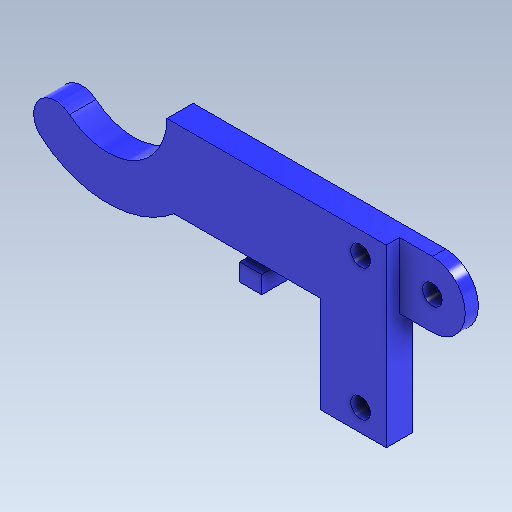
# Autodesk Inventor part: エアタンクペットボトル取付具
Saved by Autodesk Inventor 2021.3 (Build 253353010, 353A)
## iProperties
Created: 2020-02-08
Part Number: エアタンクペットボトル取付具
Material: 一般
Document SubType Name: Modeling
Designer: yuta2
Density: 1 g/cm^3
Appearance: 青 - 壁塗料 - 光沢
Author: yuta2
Autodesk Inventor part; units mm, degrees
ref_plane "YZ Plane" through (0, 0, 0) normal (1, 0, 0) x (0, 1, 0)
ref_plane "XZ Plane" through (0, 0, 0) normal (0, 1, 0) x (-1, 0, 0)
ref_plane "XY Plane" through (0, 0, 0) normal (0, 0, 1) x (1, 0, 0)
sketch "スケッチ6" plane through (0, 0, 0) normal (0, 0, 1) x (1, 0, 0)
  circle A0 centre (0, 0) radius 13.5
  circle A1 centre (0, 0) radius 23.5
  circle A2 centre (-11.8916, -14.1718) radius 5
  line L0 (0, 0) -> (-11.8916, -14.1718)
  line L1 (0, 0) -> (0, -23.5)
  line L2 (13.5, 0) -> (63.5, 0)
  line L3 (63.5, 0) -> (63.5, -18)
  line L4 (63.5, -18) -> (13.5, -18)
  line L5 (13.5, -18) -> (13.5, 0)
  line L6 (48.5, 0) -> (63.5, 0)
  line L7 (63.5, 0) -> (63.5, -40)
  line L8 (63.5, -40) -> (48.5, -40)
  line L9 (48.5, -40) -> (48.5, 0)
  point P0 (-15.1055, -18.002)
  point P1 (48.5, -18)
  point P2 (-8.6776, -10.3416)
  point P3 (23.5, 0)
  point P4 (13.3373, -19.3486)
  point P5 (13.4479, -1.1846)
  point P6 (23.5, 0)
  point P7 (15.1079, -18)
  dimension "d31" = 27
  dimension "d32" = 47
  dimension "d33" = 10
  dimension "d34" = 40
  dimension "d35" = 50
  dimension "d36" = 18
  dimension "d37" = 15
  dimension "d38" = 0
  dimension "d63" = 40
  constraints: 20 end point, 4 parallel, 2 coincident, 2 horizontal, 2 perpendicular, 2 point on line, 1 centre point, 1 vertical, 7 other
  measures "d33" diameter of A2
  measures "d34" angle of L1 L0
  measures "d35" distance of L3.end L4.end
  measures "d36" distance of L2.end L3.end
  measures "d37" distance between parallel lines of L3 L9
  measures "d38" distance between parallel lines of L2 L6
  measures "d63" distance between parallel lines of L8 L2
extrude "押し出し4" add sketch "スケッチ6" along normal blind 6 contours L5 L4 A1 L1 A0 | L2 A1 L4 L5 | A0 L1 A1 A2 | A2 | L2 L9 L4 A1 | L2 L3 L4 L9 | L4 L7 L8 L9
sketch "スケッチ9" plane through (0, 0, 6) normal (0, 0, 1) x (1, 0, 0)
  line L0 (48.5, -40) -> (63.5, -40) projected
  line L1 (63.5, 0) -> (13.5, 0) projected
  point P0 (0, 0)
  point P1 (57.6485, -5)
  point P2 (57.6485, -35)
  dimension "d54" = 5
  dimension "d64" = 5
  constraints: 1 vertical alignment
  measures "d54" distance from line of L0 point (57.649, -35)
  measures "d64" distance from line of L1 point (57.649, -5)
hole "穴4" at (57.6485, -5, 6) at (57.6485, -35, 6) direction (0, 0, -1) diameter 4.5 end through all
sketch "スケッチ10" plane through (0, 0, 0) normal (0, 0, -1) x (-1, 0, 0)
  circle A0 centre (-71, -7.5) radius 7.5
  line L0 (-63.5, -40) -> (-63.5, 0) projected
  line L1 (-63.5, 0) -> (-13.5, 0) projected
  line L2 (-63.5, -40) -> (-63.5, 0) projected
  line L3 (-71, 0) -> (-63.5, 0)
  line L4 (-63.5, 0) -> (-63.5, -15)
  line L5 (-63.5, -15) -> (-71, -15)
  line L6 (-71, -15) -> (-71, 0)
  point P0 (0, 0)
  dimension "d65" = 15
  constraints: 8 end point, 2 horizontal, 2 parallel, 1 perpendicular, 1 point on line, 1 vertical, 3 other
extrude "押し出し6" add sketch "スケッチ10" against normal blind 3
sketch "スケッチ11" plane through (0, 0, 3) normal (0, 0, 1) x (1, 0, 0)
  arc A0 (71, -15) -> (71, 0) centre (71, -7.5) ccw projected
  point P0 (0, 0)
  constraints: 1 coincident
hole "穴5" at (71, -7.5, 3) direction (0, 0, -1) diameter 4.5 end through all
sketch "スケッチ12" plane through (15.1079, -18, 0) normal (0, -1, 0) x (1, 0, 0)
  line L0 (-1.6079, 0) -> (55.8921, 0) projected
  line L1 (48.3921, 6) -> (-1.6079, 6) projected
  line L2 (20, 0) -> (15, 0)
  line L3 (15, 0) -> (15, 6)
  line L4 (15, 6) -> (20, 6)
  line L5 (20, 6) -> (20, 0)
  line L6 (0, 0) -> (0, 6) projected
  point P0 (-15.1079, 0)
  point P1 (15, 0)
  dimension "d75" = 5
  dimension "d82" = 15
  constraints: 8 end point, 2 parallel, 2 point on line, 1 horizontal, 1 perpendicular
  measures "d75" distance of L3.end L4.end
  measures "d82" distance between parallel lines of L6 L3
extrude "押し出し7" add sketch "スケッチ12" along normal blind 6 contours L3 L1 L5 L0
sketch "スケッチ13" plane through (35.1079, -18, 6) normal (1, 0, 0) x (0, 0, -1)
  line L0 (6, 0) -> (0, 0) projected
  line L1 (0, 0) -> (2, 0)
  line L2 (2, 0) -> (2, -2)
  line L3 (2, -2) -> (0, -2)
  line L4 (0, -2) -> (0, 0)
  point P0 (6, 18)
  dimension "d78" = 2
  dimension "d79" = 2
  constraints: 8 end point, 2 parallel, 1 horizontal, 1 perpendicular
  measures "d78" distance of L2.end L3.end
  measures "d79" distance of L1.end L2.end
extrude "押し出し8" cut sketch "スケッチ13" against normal blind 6
